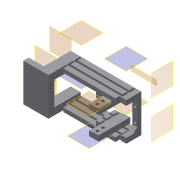
# Autodesk Inventor part: 01_Slide_camera_v1
Saved by Autodesk Inventor 2019.4 (Build 234330000, 330)
## iProperties
Created: 2021-01-21
Part Number: 01_Slide_camera_v1
Material: Generic
Document SubType Name: Modeling
Designer: diederichbenedict
Density: 1 g/cm^3
Appearance: Default
Author: diederichbenedict
Autodesk Inventor part; units mm, degrees
ref_plane "YZ Plane" through (0, 0, 0) normal (1, 0, 0) x (0, 1, 0)
ref_plane "XZ Plane" through (0, 0, 0) normal (0, 1, 0) x (-1, 0, 0)
ref_plane "XY Plane" through (0, 0, 0) normal (0, 0, 1) x (1, 0, 0)
ref_plane "Work Plane1" through (-18.4, 5, -0.4) normal (0, 0, 1) x (1, 0, 0)
ref_plane "Work Plane2" through (-62.7, -21.65, 18.5) normal (0, 0, 1) x (1, 0, 0)
ref_plane "Work Plane4" through (-69.4, 8.15, 20.5) normal (0, 0, 1) x (1, 0, 0)
sketch "Sketch5" plane through (-69.4, 8.15, 20.5) normal (0, 0, 1) x (1, 0, 0)
  line L0 (119, -34.85) -> (112.5766, -34.85)
  line L1 (112.5766, -34.85) -> (112.5766, -3.15)
  line L2 (112.5766, -3.15) -> (119, -3.15)
  line L3 (119, -3.15) -> (119, -34.85)
  line L4 (0, 0) -> (81, 0) projected
  line L5 (81, 0) -> (76, 0)
  line L6 (76, 0) -> (76, -19)
  line L7 (76, -19) -> (81, -19)
  line L8 (81, -19) -> (81, 0)
  dimension "d43" = 5
  dimension "d106" = 19
  constraints: 16 end point, 4 parallel, 2 horizontal, 2 perpendicular
  measures "d43" distance of L7.end L6.end
  measures "d106" distance between parallel lines of L7 L4
extrude "Extrusion4" add sketch "Sketch5" along normal blind 15 contours L4 L8 L7 L6
ref_plane "Work Plane5" through (-24.4, 8.15, -0.4) normal (0, -1, 0) x (1, 0, 0)
sketch "Sketch6" plane through (-24.4, 8.15, -0.4) normal (0, -1, 0) x (1, 0, 0)
  line L0 (29, 20.9) -> (-23.1996, 20.9)
  line L1 (-23.1996, 20.9) -> (-23.1996, 25.9)
  line L2 (-23.1996, 25.9) -> (29, 25.9)
  line L3 (29, 25.9) -> (29, 20.9)
  line L4 (29, 27.9) -> (-23.1996, 27.9)
  line L5 (-23.1996, 27.9) -> (-23.1996, 32.9)
  line L6 (-23.1996, 32.9) -> (29, 32.9)
  line L7 (29, 32.9) -> (29, 27.9)
  line L8 (29, 20.9) -> (31, 20.9)
  line L9 (31, 20.9) -> (31, 21.5)
  line L10 (31, 21.5) -> (29, 21.5)
  line L11 (29, 21.5) -> (29, 20.9)
  line L12 (29, 27.9) -> (31, 27.9)
  line L13 (31, 27.9) -> (31, 28.5)
  line L14 (31, 28.5) -> (29, 28.5)
  line L15 (29, 28.5) -> (29, 27.9)
  line L16 (-25.1996, 20.9) -> (-29.8432, 20.9)
  line L17 (-29.8432, 20.9) -> (-29.8432, 35.5)
  line L18 (-25.1996, 35.5) -> (-25.1996, 20.9)
  line L19 (-23.1996, 20.9) -> (-25.1996, 20.9)
  line L20 (-25.1996, 20.9) -> (-25.1996, 21.5)
  line L21 (-25.1996, 21.5) -> (-23.1996, 21.5)
  line L22 (-23.1996, 21.5) -> (-23.1996, 20.9)
  line L23 (-23.1996, 27.9) -> (-25.1996, 27.9)
  line L24 (-25.1996, 27.9) -> (-25.1996, 28.5)
  line L25 (-25.1996, 28.5) -> (-23.1996, 28.5)
  line L26 (-23.1996, 28.5) -> (-23.1996, 27.9)
  line L27 (-29.8432, 35.5) -> (-25.1996, 35.5)
  line L28 (36, 20.9) -> (31, 20.9) projected
  line L29 (31, 34.9) -> (29, 34.9)
  line L30 (29, 34.9) -> (29, 35.5)
  line L31 (29, 35.5) -> (31, 35.5)
  line L32 (31, 35.5) -> (31, 34.9)
  line L33 (29, 34.9) -> (-23.1996, 34.9)
  line L34 (-23.1996, 34.9) -> (-23.1996, 39.9)
  line L35 (-23.1996, 39.9) -> (29, 39.9)
  line L36 (29, 39.9) -> (29, 34.9)
  line L37 (-23.1996, 34.9) -> (-25.1996, 34.9)
  line L38 (-25.1996, 34.9) -> (-25.1996, 35.5)
  line L39 (-25.1996, 35.5) -> (-23.1996, 35.5)
  line L40 (-23.1996, 35.5) -> (-23.1996, 34.9)
  line L41 (31, 20.9) -> (31, 35.9) projected
  point P0 (24.4, 0.4)
  point P1 (31, 28.2)
  dimension "d30" = 5
  dimension "d32" = 5
  dimension "d33" = 0.6
  dimension "d34" = 0.6
  dimension "d40" = 2
  dimension "d41" = 2
  dimension "d48" = 2
  dimension "d49" = 2
  dimension "d55" = 2
  dimension "d56" = 0.6
  dimension "d57" = 0.6
  dimension "d91" = 0
  dimension "d112" = 2
  dimension "d113" = 0.6
  dimension "d115" = 5
  dimension "d116" = 2
  constraints: 80 end point, 19 parallel, 11 horizontal, 10 perpendicular, 6 point on line, 1 collinear, 1 midpoint
  measures "d30" distance of L0.end L1.end
  measures "d32" distance of L4.end L5.end
  measures "d33" distance between parallel lines of L10 L8
  measures "d34" distance between parallel lines of L14 L12
  measures "d40" distance between parallel lines of L3 L9
  measures "d41" distance between parallel lines of L7 L13
  measures "d48" distance between parallel lines of L18 L5
  measures "d49" distance between parallel lines of L18 L1
  measures "d55" distance between parallel lines of L4 L2
  measures "d56" distance between parallel lines of L19 L21
  measures "d57" distance between parallel lines of L25 L23
  measures "d91" distance between parallel lines of L28 L0
  measures "d112" distance of L30.end L31.end
  measures "d113" distance of L29.end L30.end
  measures "d115" distance of L33.end L34.end
  measures "d116" distance between parallel lines of L33 L6
extrude "Extrusion5" add sketch "Sketch6" along normal blind 4 contours L0 L1 L2 L3 | L3 L10 L9 L8 | L19 L18 L21 L1 | L16 L17 L27 L18 | L12 L7 L14 L13 | L18 L25 L5 L23 | L4 L5 L6 L7 | L39 L34 L37 L18 | L29 L30 L31 L32 | L34 L35 L36 L30 L33
ref_plane "Work Plane11" through (11.6, -29.85, -0.4) normal (1, 0, 0) x (0, 0, -1)
sketch "Sketch9" plane through (11.6, -29.85, -0.4) normal (1, 0, 0) x (0, 0, -1)
  line L0 (-20.9, 19) -> (-20.9, 38) projected
  line L1 (-20.9, 38) -> (-35.9, 38) projected
  line L2 (-35.9, 19) -> (-35.9, 38) projected
  line L3 (-20.9, 19) -> (-35.9, 19) projected
  line L4 (-46.9, 5) -> (-24.9, 5)
  line L5 (-24.9, 5) -> (-24.9, 29)
  line L6 (-28.9, 33) -> (-46.9, 33)
  line L7 (-46.9, 33) -> (-46.9, 5)
  line L8 (-46.9, 5) -> (-24.9, 33) construction
  line L9 (-24.9, 5) -> (-46.9, 33) construction
  line L10 (-24.9, 29) -> (-28.9, 33)
  point P0 (-0.4, 29.85)
  dimension "d107" = 22
  dimension "d108" = 28
  dimension "d109" = 4
  dimension "d110" = 4
  constraints: 14 end point, 2 midpoint, 2 parallel, 2 point on line, 1 horizontal, 1 perpendicular
  measures "d107" distance of L6.end L8.end
  measures "d108" distance of L8.end L4.end
  measures "d109" distance of L5.end L8.end
  measures "d110" distance of L6.start L8.end
extrude "Extrusion8" cut sketch "Sketch9" against normal blind 5 contours L5 L4 L7 L6 L2 L3 | L3 L2 L6 L10 L5
ref_plane "Work Plane7" through (-69.4, 8.15, -0.4) normal (0, 1, 0) x (1, 0, 0)
sketch "Sketch10" plane through (-69.4, 8.15, -0.4) normal (0, 1, 0) x (1, 0, 0)
  line L0 (58.4137, -20.9) -> (54.4137, -20.9)
  line L1 (54.4137, -20.9) -> (54.4137, -25.9)
  line L2 (54.4137, -25.9) -> (58.4137, -25.9)
  line L3 (58.4137, -25.9) -> (58.4137, -20.9)
  line L4 (58.4137, -27.9) -> (54.4137, -27.9)
  line L5 (54.4137, -27.9) -> (54.4137, -32.9)
  line L6 (54.4137, -32.9) -> (58.4137, -32.9)
  line L7 (58.4137, -32.9) -> (58.4137, -27.9)
  line L8 (58.4137, -20.9) -> (60.4137, -20.9)
  line L9 (60.4137, -20.9) -> (60.4137, -21.5)
  line L10 (60.4137, -21.5) -> (58.4137, -21.5)
  line L11 (58.4137, -21.5) -> (58.4137, -20.9)
  line L12 (58.4137, -27.9) -> (60.4137, -27.9)
  line L13 (60.4137, -27.9) -> (60.4137, -28.5)
  line L14 (60.4137, -28.5) -> (58.4137, -28.5)
  line L15 (58.4137, -28.5) -> (58.4137, -27.9)
  line L16 (19.8004, -27.9) -> (76, -27.9) projected
  line L17 (15.1568, -20.9) -> (76, -20.9) projected
  line L18 (54.4137, -34.9) -> (58.4137, -34.9)
  line L19 (58.4137, -34.9) -> (58.4137, -39.9)
  line L20 (58.4137, -39.9) -> (54.4137, -39.9)
  line L21 (54.4137, -39.9) -> (54.4137, -34.9)
  line L22 (58.4137, -34.9) -> (60.4137, -34.9)
  line L23 (60.4137, -34.9) -> (60.4137, -35.5)
  line L24 (60.4137, -35.5) -> (58.4137, -35.5)
  line L25 (58.4137, -35.5) -> (58.4137, -34.9)
  point P0 (69.4, -0.4)
  dimension "d62" = 4
  dimension "d63" = 5
  dimension "d66" = 2
  dimension "d67" = 0.6
  dimension "d68" = 0.6
  dimension "d72" = 4
  dimension "d73" = 0
  dimension "d92" = 0
  dimension "d93" = 5
  dimension "d94" = 0
  dimension "d121" = 4
  dimension "d122" = 5
  dimension "d123" = 0.6
  dimension "d124" = 2
  constraints: 48 end point, 12 parallel, 6 horizontal, 6 perpendicular, 1 point on line
  measures "d62" distance of L2.end L1.end
  measures "d63" distance of L1.end L0.end
  measures "d66" distance of L9.end L10.end
  measures "d67" distance of L8.end L9.end
  measures "d68" distance of L12.end L13.end
  measures "d72" distance between parallel lines of L7 L5
  measures "d73" distance between parallel lines of L1 L5
  measures "d92" distance between parallel lines of L16 L4
  measures "d93" distance between parallel lines of L4 L6
  measures "d94" distance between parallel lines of L17 L0
  measures "d121" distance of L19.end L20.end
  measures "d122" distance of L18.end L19.end
  measures "d123" distance of L22.end L23.end
  measures "d124" distance between parallel lines of L18 L6
extrude "Extrusion9" add sketch "Sketch10" against normal blind 9
ref_plane "Work Plane3" through (-53.4706, -12.4206, 52.3) normal (0, 0, 1) x (1, 0, 0)
ref_plane "Work Plane13" through (-69.4, -0.85, 35.5) normal (0, 0, 1) x (1, 0, 0)
sketch "Sketch11" plane through (-69.4, -0.85, 35.5) normal (0, 0, 1) x (1, 0, 0)
  line L0 (58.4137, 5) -> (58.4137, 0) projected
  line L1 (60.4137, 0) -> (58.4137, 0) projected
  line L2 (60.4137, 5) -> (60.4137, 0) projected
  spline S0 degree 3 poles (30.4003, 2.5) (53.3024, -1.5383) (73.3587, -2.9787) (96.0407, -2.7861) knots 0 0 0 0 1 1 1 1 construction
  line L3 (60.4137, 5) -> (60.4137, 0) projected
  line L4 (60.4137, 4.226) -> (70.026, 4.226)
  line L5 (70.026, 4.226) -> (70.026, -1.7861)
  line L6 (60.4137, 4.226) -> (60.4137, -1.0864)
  line L7 (58.4137, 5) -> (60.4137, 5) projected
  spline S1 degree 4 poles (60.4137, -1.0864) (61.1436, -1.1503) (61.8737, -1.212) (64.2753, -1.4077) (66.6787, -1.5798) (68.352, -1.6884) (70.026, -1.786) knots 0 0 0 0 0 0.304091 0.304091 1 1 1 1 1
  spline S2 degree 4 poles (30.5739, 3.4848) (38.7207, 2.0487) (46.9085, 0.8395) (63.2572, -0.9988) (79.6917, -1.7406) (87.8631, -1.855) (96.0322, -1.7862) knots 0 0 0 0 0 0.503132 0.503132 1 1 1 1 1
  point P0 (69.4, 0.85)
  point P1 (60.4137, -0.4862)
  point P2 (70.026, -1.1871)
  dimension "d77" = 1
  constraints: 6 end point, 3 point on line, 1 horizontal, 1 perpendicular, 1 vertical, 8 other
extrude "Extrusion10" add sketch "Sketch11" along normal up to surface (31.8 mm away) from surface at -15 contours L2 L4 L5 S2 L6
ref_plane "Work Plane12" through (-8.9863, -25.076, 52.3) normal (0, -1, 0) x (1, 0, 0)
sketch "Sketch12" plane through (-8.9863, -25.076, 52.3) normal (0, -1, 0) x (1, 0, 0)
  line L0 (0, 0) -> (9.6123, 0) projected
  line L1 (0, 0) -> (0, -21.2) projected
  line L2 (0, -21.2) -> (0, -21.8) projected
  line L3 (0, -21.8) -> (0, -28.2) projected
  line L4 (0, -28.2) -> (0, -28.8) projected
  line L5 (9.6123, -28.8) -> (0, -28.8) projected
  line L6 (9.6123, -28.8) -> (9.6123, 0) projected
  circle A0 centre (4.8062, -3.4424) radius 1.45
  circle A1 centre (4.8062, -9.262) radius 1.45
  point P0 (8.9863, -52.3)
  dimension "d78" = 2.9
  dimension "d79" = 2.9
  constraints: 2 centre point
  measures "d78" diameter of A0
  measures "d79" diameter of A1
extrude "Extrusion11" cut sketch "Sketch12" against normal through all contours A0 | A1
sketch "Sketch15" plane through (-54.2432, 8.15, 20.5) normal (-1, 0, 0) x (0, 0, 1)
  line L0 (14.6, 0) -> (0, 0) projected
  line L1 (0, 0) -> (0, -4) projected
  line L2 (14.6, -4) -> (0, -4) projected
  line L3 (14.6, 0) -> (14.6, -4) projected
  line L4 (12, -4) -> (12, -9) projected
  line L5 (0, 0) -> (12, 0)
  line L6 (12, 0) -> (12, -7)
  line L7 (12, -7) -> (0, -7)
  line L8 (0, -7) -> (0, 0)
  line L9 (7, -4.774) -> (7, -9) projected
  line L10 (7, -4.774) -> (0.6, -4.774) projected
  line L11 (0.6, -4.774) -> (0.6, -9) projected
  line L12 (0, -9) -> (0.6, -9) projected
  line L13 (0, -9.4862) -> (0, -9) projected
  line L14 (0, -9.4862) -> (31.8, -9.4862) projected
  line L15 (31.8, -9.4862) -> (31.8, -4.774) projected
  line L16 (31.8, -4.774) -> (14.6, -4.774) projected
  line L17 (7.6, -4.774) -> (7.6, -9) projected
  line L18 (7, -9) -> (7.6, -9) projected
  line L19 (12, 0) -> (32.3544, 0)
  line L20 (12, 0) -> (32.3544, 0) construction
  line L21 (32.3544, 0) -> (32.3544, -19)
  line L22 (12, -7) -> (32.9214, -7) construction
  line L23 (30.3544, -19) -> (32.3544, -19)
  line L24 (0, -19) -> (4, -19) projected
  line L25 (14, -4.774) -> (14, -9) projected
  line L26 (14, -4.774) -> (7.6, -4.774) projected
  line L27 (14.6, -4.774) -> (14.6, -9) projected
  line L28 (14, -9) -> (14.6, -9) projected
  line L29 (12, -7) -> (26.535, -7)
  line L30 (26.535, -7) -> (26.535, -19)
  line L31 (12, -4) -> (12, -9) projected
  line L32 (26.535, -19) -> (32.3544, -19)
  point P0 (-20.5, -8.15)
  dimension "d101" = 7
  dimension "d102" = 0
  dimension "d111" = 0
  dimension "d125" = 2
  constraints: 24 end point, 4 horizontal, 4 parallel, 2 perpendicular, 1 collinear, 1 vertical, 2 other
  measures "d101" distance of L5.end L6.end
  measures "d102" distance between parallel lines of L19 L20
  measures "d111" distance between parallel lines of L23 L24
  measures "d125" distance from line of L23.start L21
extrude "Extrusion14" add sketch "Sketch15" along normal mid plane 10 contours L3 L2 L6 L0 | L19 L21 L23 L32 L30 L14 L15 L16 L27 L29 L25 L26 L4 L2 L3 | L6 L2 L1 L0 | L4 L26 L17 L7 L9 L10 L11 L8 L2 | L26 L25 L29 L4 | L4 L7 L17 L26 | L11 L10 L9 L7 | L30 L29 L27 L16 L15 L14
sketch "Sketch16" plane through (6.6, -10.85, 24.5) normal (0, 0, 1) x (1, 0, 0)
  line L0 (5, 0) -> (0, 0) projected
  line L1 (5, 10) -> (5, 0) projected
  line L2 (5, 10) -> (0, 10) projected
  line L3 (0, 0) -> (0, 10) projected
  circle A0 centre (2.5, 7) radius 1.45
  point P0 (-6.6, 10.85)
  dimension "d117" = 2.9
  dimension "d118" = 7
  constraints: 1 centre point
  measures "d117" diameter of A0
  measures "d118" distance from line of A0.centre L0
extrude "Extrusion15" cut sketch "Sketch16" against normal blind 10 contours A0
mirror "Mirror2" about plane through (6.6, -10.85, 20.5) normal (0, -1, 0) of "Extrusion4", "Extrusion5", "Extrusion8", "Extrusion9", "Extrusion10", "Extrusion11", "Extrusion14", "Extrusion15"
sketch "Sketch18" plane through (4.6, -29.85, 35.1) normal (0, -1, 0) x (1, 0, 0)
  line L0 (-79, 12.4) -> (-65, 12.4)
  line L1 (-63.8432, 17.7544) -> (-53.8432, 17.7544) projected
  line L2 (-63.8432, 17.7544) -> (-63.8432, -14.6) projected
  line L3 (-63.8432, 17.7544) -> (-79, 17.7544)
  line L4 (-79, 17.7544) -> (-79, 12.4)
  line L5 (-79, 12.4) -> (-63.8432, 12.4)
  line L6 (-63.8432, 12.4) -> (-63.8432, 17.7544)
  point P0 (-4.6, -35.1)
  constraints: 10 end point, 2 horizontal, 2 parallel, 1 perpendicular, 2 other
extrude "Extrusion17" add sketch "Sketch18" against normal up to surface (38 mm away)
ref_plane "Work Plane14" through (-24.4, -29.85, -0.4) normal (0, -1, 0) x (1, 0, 0)
ref_plane "Work Plane15" through (-69.4, -29.85, -0.4) normal (0, 1, 0) x (1, 0, 0)
ref_plane "Work Plane16" through (11.6, 8.15, -0.4) normal (-1, 0, 0) x (0, 0, -1)
ref_plane "Work Plane17" through (-8.9863, 3.376, 52.3) normal (0, -1, 0) x (1, 0, 0)
ref_plane "Work Plane18" through (-69.4, -20.85, 35.5) normal (0, 0, -1) x (1, 0, 0)
ref_plane "Work Plane19" through (-53.4706, -9.2794, 52.3) normal (0, 0, -1) x (1, 0, 0)
equation "\"d110\" = d109"
body "Solid1"
